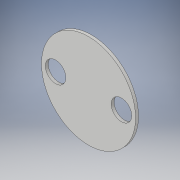
# Autodesk Inventor part: main_plate
Saved by Autodesk Inventor 2019.3 (Build 233278000, 278)
## iProperties
Created: 2019-04-09
Part Number: main_plate
Material: Generic
Document SubType Name: Modeling
Designer: Connor
Density: 1 g/cm^3
Appearance: Default
Author: Connor
Autodesk Inventor part; units mm, degrees
ref_plane "YZ Plane" through (0, 0, 0) normal (1, 0, 0) x (0, 1, 0)
ref_plane "XZ Plane" through (0, 0, 0) normal (0, 1, 0) x (-1, 0, 0)
ref_plane "XY Plane" through (0, 0, 0) normal (0, 0, 1) x (1, 0, 0)
sketch "Sketch1" plane through (0, 0, 0) normal (0, 0, 1) x (1, 0, 0)
  circle A0 centre (0, 0) radius 50.8
  circle A1 centre (-35.56, 0) radius 11.1125
  circle A2 centre (35.56, 0) radius 11.1125
  line L0 (-35.56, 0) -> (0, 0) construction
  line L1 (0, 0) -> (35.56, 0) construction
  dimension "d0" = 22.225
  dimension "d1" = 22.225
  dimension "d2" = 71.12
  dimension "d3" = 101.6
  constraints: 4 end point, 3 centre point, 2 collinear, 2 horizontal alignment, 1 coincident, 1 horizontal
  measures "d0" diameter of A1
  measures "d1" diameter of A2
  measures "d2" distance of L1.end L0.start
  measures "d3" diameter of A0
extrude "Extrusion1" add sketch "Sketch1" along normal blind 3.175
body "Solid1"
